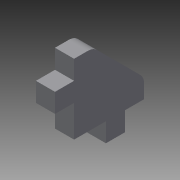
# Autodesk Inventor part: Endplate_B Support
Saved by Autodesk Inventor 2015 (Build 190159000, 159)
## iProperties
Created: 2013-05-28
Part Number: Endplate_B Support
Material: Generic
Document SubType Name: Modeling
Designer: Eric
Density: 1 g/cm^3
Appearance: Default
Author: Eric
Autodesk Inventor part; units mm, degrees
ref_plane "YZ Plane" through (0, 0, 0) normal (1, 0, 0) x (0, 1, 0)
ref_plane "XZ Plane" through (0, 0, 0) normal (0, 1, 0) x (-1, 0, 0)
ref_plane "XY Plane" through (0, 0, 0) normal (0, 0, 1) x (1, 0, 0)
sketch "Sketch1" plane through (0, 0, 0) normal (1, 0, 0) x (0, 1, 0)
  line L0 (0, 0) -> (0, 5)
  line L1 (0, 5) -> (-3, 5)
  line L2 (-3, 5) -> (-3, 8)
  line L3 (-3, 8) -> (0, 8)
  line L4 (0, 8) -> (0, 11)
  line L5 (0, 11) -> (2.1716, 11)
  line L6 (11, 0) -> (8, 0)
  line L7 (8, 0) -> (8, -3)
  line L8 (8, -3) -> (5, -3)
  line L9 (5, -3) -> (5, 0)
  line L10 (5, 0) -> (0, 0)
  line L11 (11, 0) -> (11, 2.1716)
  line L12 (10.4142, 3.5858) -> (3.5858, 10.4142)
  arc A0 (3.5858, 10.4142) -> (2.1716, 11) centre (2.1716, 9) ccw
  arc A1 (11, 2.1716) -> (10.4142, 3.5858) centre (9, 2.1716) ccw
  point P0 (3, 11)
  point P1 (11, 3)
  dimension "d0" = 5
  dimension "d1" = 3
  dimension "d2" = 3
  dimension "d3" = 5
  dimension "d4" = 3
  dimension "d5" = 3
  dimension "d6" = 3
  dimension "d7" = 3
  dimension "d8" = 3
  dimension "d9" = 3
  dimension "d10" = 3
  dimension "d11" = 3
  dimension "d14" = 2
  constraints: 26 end point, 8 parallel, 4 point on circle, 4 point on line, 4 tangent, 2 centre point, 2 perpendicular, 1 collinear, 1 equal radius, 1 vertical
  measures "d0" distance of L9.end L0.start
  measures "d1" distance of L7.end L8.end
  measures "d2" distance of L6.start L6.end
  measures "d3" distance of L0.start L0.end
  measures "d4" distance of L1.end L2.end
  measures "d5" distance of L3.end L4.end
  measures "d6" distance of L0.end L1.end
  measures "d7" distance of L8.end L9.end
  measures "d8" distance of L6.end L7.end
  measures "d9" distance of L6.start point (11, 3)
  measures "d10" distance of L4.end point (3, 11)
  measures "d11" distance of L2.end L3.end
  measures "d14" radius of A0
extrude "Extrusion1" add sketch "Sketch1" along normal blind 3
body "Solid1"
